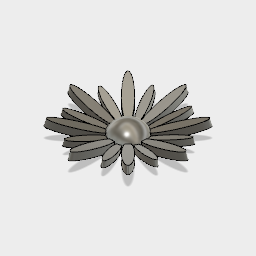
花 v1 (Autodesk Fusion 360 design; units mm, degrees)
Autodesk Fusion 360 part; units mm, degrees
note: some values were not read from the file. Set by a fixed rule: which face or edge a step refers to.
sketch "草图1" plane through (0, 0, 0) normal (0, 1, 0) x (1, 0, 0)
  ellipse E0 centre (0, 0) end of major axis (-10, 0) minor radius 2
  line L0 (10, 0) -> (-10, 0)
  line L1 (0, 2) -> (0, -2)
  dimension "d1" = 10
  dimension "d2" = 4
  measures "d1" distance of E0
extrude "拉伸1" add sketch "草图1" along normal blind 3 makes body 1
move_body "移动1" bodies 1 to x (0.965926, 0.258819, 0) y (-0.258819, 0.965926, 0) z (0, 0, 1) at (-0.2161, 2.5683, 0)
move_face "MoveFace1" to x (1, 0, 0) y (0, 1, 0) z (0, 0, 1) at (22, 29, 22) 1 faces at (-3.3539, 2.7628, -1.9091) on bodies 1
move_face "MoveFace2" to x (1, 0, 0) y (0, 1, 0) z (0, 0, 1) at (-14, 30, 0) 1 faces at (25.672, 11.5756, 23.9798) on bodies 1
move_face "MoveFace3" to x (1, 0, 0) y (0, 1, 0) z (0, 0, 1) at (-10, 28, 0) 1 faces at (18.6014, 9.681, 23.9091) on bodies 1
move_face "MoveFace4" to x (1, 0, 0) y (0, 1, 0) z (0, 0, 1) at (0, 28, 0) 1 faces at (16.5301, 8.0907, 23.9091) on bodies 1
move_body "移动2" bodies 1 to x (1, 0, 0) y (0, 1, 0) z (0, 0, 1) at (-8, 1, 0)
move_body "移动3" bodies 1 to x (1, 0, 0) y (0, 1, 0) z (0, 0, 1) at (0, -8, 0)
move_face "MoveFace5" by (0, 0, -28) 1 faces at (15.4843, 5.0246, 21.4019) on bodies 1
move_body "移动4" bodies 1 to x (1, 0, 0) y (0, 1, 0) z (0, 0, 1) at (0, 0, -22)
move_body "移动5" bodies 1 to x (1, 0, 0) y (0, 1, 0) z (0, 0, 1) at (-3, 0, 0)
pattern_circular "C-阵列1" count 8 over 360 about axis through (0, 1.75, 0) along (0, 1, 0) of bodies 1 makes body 2 at (8.9538, 2.1269, -9.7997) makes body 3 at (0.5981, 3.4169, -18.0751) makes body 4 at (-9.7997, 2.1269, -8.9538) makes body 5 at (-18.0751, 3.4169, -0.5981) makes body 6 at (-8.9538, 2.1269, 9.7997) makes body 7 at (-0.5981, 3.4169, 18.0751) makes body 8 at (9.7997, 2.1269, 8.9538)
copy_body "复制和粘贴实体1" bodies 1 makes body 9
move_body "移动6" bodies 9 to x (1, 0, 0) y (0, 1, 0) z (0, 0, 1) at (11.6004, 6.7091, -4.3469)
scale "缩放1" factor 0.8 about (36.1511, 14.9669, -4.3469) bodies 9
move_body "移动7" bodies 9 to x (0.909133, -0.016022, -0.416198) y (-0.016022, 0.997175, -0.073387) z (0.416198, 0.073387, 0.906308) at (-13.1687, -12.0942, 11.1197)
move_body "移动8" bodies 9 to x (1, 0, 0) y (0, 1, 0) z (0, 0, 1) at (1.479, 4.6038, 0.3064)
pattern_circular "C-阵列2" count 8 over 360 about axis through (0, 1.75, 0) along (0, 1, 0) of bodies 9 makes body 10 at (4.1176, 1.7547, -11.1498) makes body 11 at (-4.9725, 1.7547, -10.7957) makes body 12 at (-11.1498, 1.7547, -4.1176) makes body 13 at (-10.7957, 1.7547, 4.9725) makes body 14 at (-6.2897, 2.7923, 14.4694) makes body 15 at (5.7839, 2.7923, 14.679) makes body 16 at (11.1498, 1.7547, 4.1176)
sphere "球体基本要素1" add diameter 4 placed x (0, 0, -1) y (0, 1, 0) z (1, 0, 0) at (0, 0, 0) separate body makes body 17
delete_face "删除面1" 1 faces at (-0.4256, 0.4728, -1.8961) on bodies 17
sphere "球体基本要素2" add diameter 15 placed x (1, 0, 0) y (0, 1, 0) z (0, 0, 1) at (0, 0, 0) bodies 1 2 3 4 5 6 7 8 9 10 11 12 13 14 15 16
move_body "移动9" bodies 1 to x (1, 0, 0) y (0, 1, 0) z (0, 0, 1) at (0, 15, 0)
box "长方体基本要素4" cut length 53 width 104 height 16 placed x (0, 0, -1) y (-1, 0, 0) z (0, 1, 0) at (47, 0, 20) bodies 1
